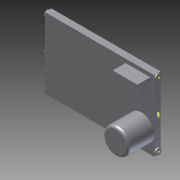
# Autodesk Inventor part: ESC
Saved by Autodesk Inventor 2011 SP1 (Build 150282100, 282)
## iProperties
Created: 2011-06-12
Part Number: ESC
Document SubType Name: Modeling
Designer: Andrew G. Meyer
Mass: 1.04769 g
Surface Area: 12.8255 cm^2
Volume: 1.04769 cm^3
Density: 1 g/cm^3
Author: Andrew G. Meyer
Autodesk Inventor part; units mm, degrees
ref_plane "YZ Plane" through (0, 0, 0) normal (1, 0, 0) x (0, 1, 0)
ref_plane "XZ Plane" through (0, 0, 0) normal (0, 1, 0) x (-1, 0, 0)
ref_plane "XY Plane" through (0, 0, 0) normal (0, 0, 1) x (1, 0, 0)
sketch "Sketch1" plane through (0, 0, 0) normal (0, 0, 1) x (1, 0, 0)
  line L0 (-19.520958, 8.240943) -> (7.466542, 8.240943)
  line L1 (7.466542, 8.240943) -> (7.466542, -9.221557)
  line L2 (7.466542, -9.221557) -> (-19.520958, -9.221557)
  line L3 (-19.520958, -9.221557) -> (-19.520958, 8.240943)
  point P0 (0, 0)
  dimension "d0" = 17.4625
  dimension "d1" = 26.9875
  constraints: 8 end point, 2 parallel, 1 horizontal, 1 perpendicular
  measures "d0" distance of L2.end L0.start
  measures "d1" distance of L0.start L0.end
extrude "Extrusion1" add sketch "Sketch1" along normal blind 1.5875
sketch "Sketch2" plane through (0, 0, 1.5875) normal (0, 0, 1) x (1, 0, 0)
  line L0 (7.466542, 8.240943) -> (7.466542, -9.221557)
  line L1 (7.466542, -9.221557) -> (-19.520958, -9.221557)
  circle A0 centre (4.291542, -4.459057) radius 3.175
  point P0 (0, 0)
  dimension "d4" = 4.7625
  dimension "d5" = 6.35
  constraints: 1 centre point, 1 tangent
  measures "d4" distance from line of L1 A0.centre
  measures "d5" diameter of A0
extrude "Extrusion2" add sketch "Sketch2" along normal blind 6.35
fillet "Fillet1" radius 0.635 1 edges at (1.1165, -4.4591, 7.9375)
sketch "Sketch3" plane through (0, 0, 1.5875) normal (0, 0, 1) x (1, 0, 0)
  line L0 (0.379367, 7.296145) -> (6.490253, 7.296145)
  line L1 (6.490253, 7.296145) -> (6.490253, 2.269448)
  line L2 (6.490253, 2.269448) -> (0.379367, 2.269448)
  line L3 (0.379367, 2.269448) -> (0.379367, 7.296145)
  point P0 (0, 0)
  constraints: 8 end point, 2 parallel, 1 horizontal, 1 perpendicular
extrude "Extrusion3" add sketch "Sketch3" along normal blind 3.175
sketch "Sketch4" plane through (7.466542, -9.221557, 0) normal (1, 0, 0) x (0, 0, -1)
  line L0 (-1.5875, 17.4625) -> (-1.5875, 4.7625)
  line L1 (-1.5875, 4.7625) -> (-1.5875, 0)
  line L2 (0, 0) -> (-1.5875, 0)
  line L3 (0, 17.4625) -> (0, 0)
  line L4 (0, 17.4625) -> (-1.5875, 17.4625)
  circle A0 centre (-0.79375, 16.66875) radius 0.79375
  circle A1 centre (-0.79375, 0.79375) radius 0.79375
  circle A2 centre (-0.79375, 8.73125) radius 0.15875
  circle A3 centre (-0.79375, 9.04875) radius 0.15875
  circle A4 centre (-0.79375, 8.41375) radius 0.15875
  line L5 (-0.79375, 0.79375) -> (-0.79375, 16.66875) construction
  line L6 (-0.79375, 0.79375) -> (-0.79375, 8.73125) construction
  line L7 (-0.79375, 8.73125) -> (-0.79375, 16.66875) construction
  point P0 (0, 9.221557)
  dimension "d11" = 0.3175
  constraints: 8 tangent, 6 end point, 5 centre point, 3 collinear, 2 equal radius, 2 point on line, 1 midpoint, 1 perpendicular
  measures "d11" diameter of A2
extrude "Extrusion4" add sketch "Sketch4" along normal blind 0.254 contours A0 | A1 | A2 | A4 | A3
sketch "Sketch5" plane through (-19.520958, -9.221557, 0) normal (-1, 0, 0) x (0, 0, 1)
  line L0 (1.5875, 0) -> (1.5875, 17.4625)
  line L1 (0, 17.4625) -> (1.5875, 17.4625)
  line L2 (0, 0) -> (0, 17.4625)
  line L3 (0, 0) -> (1.5875, 0)
  circle A0 centre (0.79375, 16.66875) radius 0.79375
  circle A1 centre (0.79375, 8.73125) radius 0.79375
  circle A2 centre (0.79375, 0.79375) radius 0.79375
  line L4 (0.79375, 16.66875) -> (0.79375, 8.73125) construction
  line L5 (0.79375, 0.79375) -> (0.79375, 8.73125) construction
  point P0 (0, 9.221557)
  constraints: 8 tangent, 4 end point, 3 centre point, 1 collinear, 1 parallel, 1 perpendicular
extrude "Extrusion5" add sketch "Sketch5" along normal blind 0.254 contours A2 | A1 | A0
sketch "Sketch6" plane through (7.720542, -8.427807, 0.79375) normal (1, 0, 0) x (0, 0, -1)
  circle A0 centre (0, 0) radius 0.79375 construction
sketch "Sketch7" plane through (7.720542, -0.172807, 0.79375) normal (1, 0, 0) x (0, 0, -1)
  circle A0 centre (0, 0) radius 0.15875 construction
  point P0 (0, -0.15875)
  constraints: 1 vertical alignment
sketch "Sketch8" plane through (7.720542, -9.221557, 0) normal (1, 0, 0) x (0, 0, -1)
  arc A0 (-0.79375, 8.5725) -> (-0.79375, 8.89) centre (-0.79375, 8.73125) ccw construction
sketch "Sketch9" plane through (7.720542, -0.807807, 0.79375) normal (1, 0, 0) x (0, 0, -1)
  circle A0 centre (0, 0) radius 0.15875 construction
  point P0 (0, 0.15875)
  constraints: 1 vertical alignment
sketch "Sketch10" plane through (-19.774958, 7.447193, 0.79375) normal (-1, 0, 0) x (0, 0, 1)
  circle A0 centre (0, 0) radius 0.79375 construction
sketch "Sketch11" plane through (-19.774958, -0.490307, 0.79375) normal (-1, 0, 0) x (0, 0, 1)
  circle A0 centre (0, 0) radius 0.79375 construction
sketch "Sketch12" plane through (-19.774958, -8.427807, 0.79375) normal (-1, 0, 0) x (0, 0, 1)
  circle A0 centre (0, 0) radius 0.79375 construction
body "Solid1"
